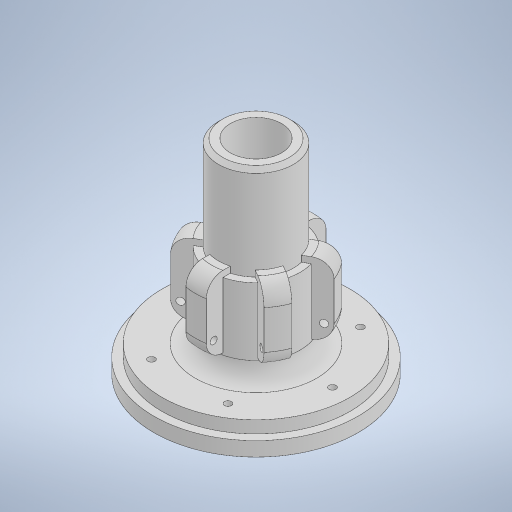
# Autodesk Inventor part: Soporte
Saved by Autodesk Inventor 2024.3 (Build 283343000, 343)
## iProperties
Created: 2024-11-12
Part Number: Soporte
Material: Generic
Document SubType Name: Modeling
Designer: j.santaa
Density: 1 g/cm^3
Appearance: Default
Mass: 170.581 g
Surface Area: 426.199 cm^2
Volume: 170.581 cm^3
Author: j.santaa
Autodesk Inventor part; units mm, degrees
ref_plane "YZ Plane" through (0, 0, 0) normal (1, 0, 0) x (0, 1, 0)
ref_plane "XZ Plane" through (0, 0, 0) normal (0, 1, 0) x (-1, 0, 0)
ref_plane "XY Plane" through (0, 0, 0) normal (0, 0, 1) x (1, 0, 0)
sketch "Sketch1" plane through (0, 0, 0) normal (0, 0, 1) x (1, 0, 0)
  circle A0 centre (0, 0) radius 50
  circle A1 centre (0, 0) radius 12.5
  circle A2 centre (0, 0) radius 18.3
  line L0 (-15.5, -15.5) -> (15.5, -15.5) construction
  line L1 (15.5, -15.5) -> (15.5, 15.5) construction
  line L2 (15.5, 15.5) -> (-15.5, 15.5) construction
  line L3 (-15.5, 15.5) -> (-15.5, -15.5) construction
  line L4 (-15.5, -15.5) -> (15.5, 15.5) construction
  line L5 (15.5, -15.5) -> (-15.5, 15.5) construction
  dimension "Diametro" = 100
  dimension "d1" = 25
  dimension "d2" = 5.8
  dimension "d8" = 31
  constraints: 12 end point, 6 coincident, 3 centre point, 2 midpoint, 2 parallel, 2 perpendicular, 1 horizontal
  measures "Diametro" diameter of A0
  measures "d1" diameter of A1
  measures "d2" radial gap between concentric circles of A1 A2
  measures "d8" distance of L0.end L1.end
extrude "Extrusion1" add sketch "Sketch1" along normal blind 7 contours A0 | A2
extrude "Extrusion2" add sketch "Sketch1" along normal blind 100 contours A2
ref_plane "Work Plane1" through (0, 0, 22) normal (0, 0, 1) x (1, 0, 0)
sketch "Sketch2" plane through (0, 0, 22) normal (0, 0, 1) x (1, 0, 0)
  arc A0 (5, 29.3268) -> (-5, 29.3268) centre (0, 0) ccw
  line L0 (5, 29.3268) -> (5, 17.6037)
  line L1 (-5, 29.3268) -> (-5, 17.6037)
  line L2 (0, -70) -> (0, 70) projected
  circle A1 centre (0, 0) radius 18.3 projected
  point P0 (0, 29.75)
  dimension "d24" = 10
  dimension "d25" = 29.75
  dimension "Dedos" = 10
  constraints: 5 point on circle, 4 end point, 1 centre point, 1 coincident, 1 vertical alignment, 1 other
  measures "d24" distance of L1.start L0.start
  measures "d25" distance of point (0, 0) point (0, 29.75)
  measures "Dedos" distance of L0.end L1.end
extrude "Extrusion3" add sketch "Sketch2" along normal blind 15 contours L0 A1 L2 A0 | L2 A1 L1 A0
sketch "Sketch3" plane through (0, 0, 0) normal (1, 0, 0) x (0, 1, 0)
  line L0 (29.75, 37) -> (29.3268, 37) projected
  line L1 (17.6037, 22) -> (18.3, 22) projected
  line L2 (29.75, 22) -> (29.75, 37) projected
  line L3 (17.6037, 22) -> (17.6037, 37) projected
  circle A0 centre (25.74, 29.5) radius 1.5
  line L4 (0, -7.4) -> (0, 44.4) projected
  point P0 (0, 0)
  point P1 (29.75, 29.5)
  dimension "d31" = 3
  dimension "d92" = 25.74
  constraints: 1 centre point, 1 coincident, 1 horizontal alignment, 1 midpoint
  measures "d31" diameter of A0
  measures "d92" distance from line of L4 A0.centre
fillet "Fillet2" radius 8 1 edges at (0, 29.75, 22)
pattern_circular "Circular Pattern1" count 6 over 360 about axis through (0, 0, 0) along (0, 0, 1) of "Fillet2", "Extrusion3"
ref_plane "Plano de trabajo2" through (0, 0, 54) normal (0, 0, 1) x (1, 0, 0)
sketch "Boceto4" plane through (0, 0, 54) normal (0, 0, 1) x (1, 0, 0)
  circle A0 centre (0, 0) radius 21.75
  circle A1 centre (0, 0) radius 18.3 projected
  line L0 (4, -23.75) -> (4, -26.75) projected
  dimension "d54" = 43.5
  constraints: 1 centre point, 1 coincident
  measures "d54" diameter of A0
extrude "Extrusión5" add sketch "Boceto4" against normal up to surface (47 mm away)
sketch "Boceto5" plane through (0, 0, 37) normal (0, 0, 1) x (1, 0, 0)
  arc A0 (-5, -21.1675) -> (5, -21.1675) centre (0, 0) ccw projected
  line L0 (-5, -21.1675) -> (-5, -29.3268) projected
  arc A1 (-5, -29.3268) -> (5, -29.3268) centre (0, 0) ccw projected
  line L1 (5, -29.3268) -> (5, -21.1675) projected
  circle A2 centre (0, 0) radius 18.3 projected
  line L2 (5, -21.1675) -> (5, -17.6037)
  line L3 (-5, -21.1675) -> (-5, -17.6037)
  constraints: 4 end point, 2 point on circle, 1 parallel, 1 vertical
extrude "Extrusión6" add sketch "Boceto5" along normal blind 20 contours L3 A2 L2 A0 | A0 L1 A1 L0
fillet "Empalme4" radius 8 1 edges at (0, -29.75, 57)
pattern_circular "Patrón circular2" count 6 over 360 about axis through (0, 0, 54) along (0, 0, -1) of "Extrusión6", "Empalme4"
chamfer "Chaflán1" distance 2 angle 45 1 edges at (-18.3, 0, 100)
sketch "Boceto6" plane through (0, 0, 7) normal (0, 0, 1) x (1, 0, 0)
  circle A0 centre (0, 0) radius 50 projected
  arc A1 (5, -21.1675) -> (15.8316, -14.9139) centre (0, 0) ccw construction
  line L0 (0, 0) -> (18.75, -32.476) construction
  arc A2 (5, -21.1675) -> (15.8316, -14.9139) centre (0, 0) ccw construction
  point P0 (20.8316, -6.2536)
  point P1 (20.8316, 6.2536)
  point P2 (37.5, 0)
  point P3 (18.75, 32.476)
  point P4 (-18.75, 32.476)
  point P5 (-37.5, 0)
  point P6 (-18.75, -32.476)
  point P7 (10.875, -18.8361)
  dimension "d73" = 360
  dimension "d91" = 37.5
  constraints: 2 end point, 1 point on circle, 1 point on line, 7 other
  measures "d91" distance of L0.start L0.end
sketch "Boceto8" plane through (0, 0, 7) normal (0, 0, 1) x (1, 0, 0)
  circle A0 centre (0, 0) radius 21.75 projected
  circle A1 centre (0, 0) radius 50 projected
  circle A2 centre (0, 0) radius 46
  dimension "Espesor" = 4
  constraints: 1 centre point, 1 coincident
  measures "Espesor" radial gap between concentric circles of A2 A1
extrude "Extrusión8" add sketch "Boceto8" along normal blind 6 contours A2
fillet "Empalme6" radius 8 1 edges at (-21.75, 0, 13)
sketch "Boceto9" plane through (5, 17.8574, 54) normal (1, 0, 0) x (0, -1, 0)
  point P0 (-7.8826, 24.5)
hole "Agujero4" at (5, 25.74, 29.5) direction (-1, 0, 0) diameter 3.4 depth 10 tip angle 118 clearance for "Tornillo de cabeza plana avellanada ISO 2009/7046" size "M3" standard "ISO"
pattern_circular "Patrón circular3" count 6 over 360 about axis through (0, 0, 54) along (0, 0, -1) of "Agujero4"
sketch "Boceto10" plane through (0, 0, 0) normal (0, 0, -1) x (-1, 0, 0)
  line L0 (18.9835, 10.9602) -> (10.9602, -18.9835) construction
  line L1 (10.9602, -18.9835) -> (-18.9835, -10.9602) construction
  line L2 (-18.9835, -10.9602) -> (-10.9602, 18.9835) construction
  line L3 (-10.9602, 18.9835) -> (18.9835, 10.9602) construction
  line L4 (18.9835, 10.9602) -> (-18.9835, -10.9602) construction
  line L5 (10.9602, -18.9835) -> (-10.9602, 18.9835) construction
  circle A0 centre (-18.75, 32.476) radius 1.7 projected
  line L6 (-10.9602, 18.9835) -> (-18.75, 32.476) construction
  circle A1 centre (18.9835, 10.9602) radius 3.75
  circle A2 centre (10.9602, -18.9835) radius 3.75
  circle A3 centre (-18.9835, -10.9602) radius 3.75
  circle A4 centre (-10.9602, 18.9835) radius 3.75
  point P0 (0, 0)
  dimension "d97" = 31
  dimension "d98" = 7.5
  constraints: 14 end point, 4 centre point, 4 coincident, 3 equal radius, 2 midpoint, 2 parallel, 2 perpendicular, 1 collinear
  measures "d97" distance of L0.end L1.end
  measures "d98" diameter of A1
extrude "Extrusión9" cut sketch "Boceto10" against normal blind 4 contours A1 | A2 | A3 | A4
sketch "Boceto11" plane through (0, 0, 0) normal (0, 0, -1) x (-1, 0, 0)
  line L0 (0, 0) -> (0, 37.5) construction
  point P0 (0, 37.5)
  point P1 (-32.476, 18.75)
  point P2 (-32.476, -18.75)
  point P3 (0, -37.5)
  point P4 (32.476, -18.75)
  point P5 (32.476, 18.75)
  dimension "d119" = 37.5
  dimension "d122" = 360
  constraints: 2 end point, 1 coincident, 1 vertical, 7 other
  measures "d119" distance of point (0, 37.5) L0.start
hole "Agujero5" at (0, 37.5, 0) at (-32.476, 18.75, 0) at (-32.476, -18.75, 0) at (0, -37.5, 0) at (32.476, -18.75, 0) at (32.476, 18.75, 0) direction (0, 0, 1) diameter 2.459 depth 9 tip angle 120 thread size "M3x0.5" class "6H" standard "ANSI Metric M Profile"
sketch "Boceto12" plane through (0, 0, 13) normal (0, 0, 1) x (1, 0, 0)
  line L0 (0, 0) -> (18.75, -32.476) construction
  line L1 (0, 70) -> (0, -70) projected
  point P0 (37.5, 0)
  point P1 (18.75, 32.476)
  point P2 (-18.75, 32.476)
  point P3 (-37.5, 0)
  point P4 (-18.75, -32.476)
  dimension "d106" = 30
  dimension "d107" = 37.5
  dimension "d110" = 360
  constraints: 2 end point, 7 other
  measures "d106" angle of L1 L0
  measures "d107" distance of L0.start L0.end
hole "Agujero6" at (18.75, -32.476, 13) at (37.5, 0, 13) at (18.75, 32.476, 13) at (-18.75, 32.476, 13) at (-37.5, 0, 13) at (-18.75, -32.476, 13) direction (0, 0, -1) diameter 3.4 end through all clearance for "Tornillo de cabeza plana avellanada ISO 2009/7046" size "M3" standard "ISO"
sketch "Boceto13" plane through (0, 0, 13) normal (0, 0, 1) x (1, 0, 0)
  point P0 (0, 0)
equation "\"d24\" = Dedos"
equation "\"d91\" = 0.375 * Diametro"
body "Solid1"
